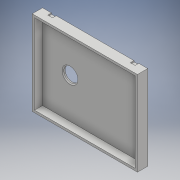
# Autodesk Inventor part: Bottom Roof
Saved by Autodesk Inventor 2017 (Build 210142000, 142)
## iProperties
Created: 2018-02-08
Part Number: Bottom Roof
Material: Generic
Document SubType Name: Modeling
Designer: Arjuna
Density: 1 g/cm^3
Appearance: Default
Author: Arjuna
## iProperties of the stored document Bottom Roof_3DPrint.ipt
Created: 2018-03-29
Part Number: Bottom Roof_3DPrint
Material: Generic
Document SubType Name: Modeling
Designer: Arjuna
Density: 1 g/cm^3
Appearance: Default
Author: Arjuna
Autodesk Inventor part; units mm, degrees
ref_plane "YZ Plane" through (0, 0, 0) normal (1, 0, 0) x (0, 1, 0)
ref_plane "XZ Plane" through (0, 0, 0) normal (0, 1, 0) x (-1, 0, 0)
ref_plane "XY Plane" through (0, 0, 0) normal (0, 0, 1) x (1, 0, 0)
sketch "Sketch1" plane through (0, 0, 0) normal (0, 1, 0) x (-1, 0, 0)
  line L0 (115, 92.5) -> (-115, 92.5)
  line L1 (-115, 92.5) -> (-115, -92.5)
  line L2 (-115, -92.5) -> (115, -92.5)
  line L3 (115, -92.5) -> (115, 92.5)
  point P0 (0, 0)
  dimension "d0" = 230
  dimension "d1" = 185
  dimension "d2" = 115
  dimension "d3" = 92.5
  constraints: 8 end point, 2 parallel, 1 horizontal, 1 perpendicular
  measures "d0" distance between parallel lines of L1 L3
  measures "d1" distance between parallel lines of L2 L0
  measures "d2" distance from line of point (0, 0) L3
  measures "d3" distance from line of point (0, 0) L2
extrude "Extrusion1" add sketch "Sketch1" along normal blind 5
sketch "Sketch2" plane through (0, 0, 0) normal (0, -1, 0) x (1, 0, 0)
  line L0 (110, 87.5) -> (-110, 87.5)
  line L1 (-110, 87.5) -> (-110, -87.5)
  line L2 (-110, -87.5) -> (110, -87.5)
  line L3 (110, -87.5) -> (110, 87.5)
  line L4 (-115, 92.5) -> (115, 92.5) projected
  line L5 (-115, -92.5) -> (-115, 92.5) projected
  line L6 (115, -92.5) -> (-115, -92.5) projected
  line L7 (115, 92.5) -> (115, -92.5) projected
  line L8 (115, 92.5) -> (-115, 92.5)
  line L9 (-115, 92.5) -> (-115, -92.5)
  line L10 (-115, -92.5) -> (115, -92.5)
  line L11 (115, -92.5) -> (115, 92.5)
  point P0 (0, 0)
  dimension "d109" = 5
  dimension "d110" = 5
  dimension "d111" = 5
  dimension "d112" = 5
  constraints: 16 end point, 4 parallel, 2 horizontal, 2 perpendicular
  measures "d109" distance between parallel lines of L2 L6
  measures "d110" distance between parallel lines of L1 L5
  measures "d111" distance between parallel lines of L4 L0
  measures "d112" distance between parallel lines of L7 L3
extrude "Extrusion2" add sketch "Sketch2" along normal blind 17.5
sketch "Sketch3" plane through (0, 5, 0) normal (0, 1, 0) x (1, 0, 0)
  circle A0 centre (-50, 0) radius 15.5
  point P0 (0, 0)
  dimension "d12" = 31
  dimension "d13" = 50
  constraints: 1 centre point
  measures "d12" diameter of A0
  measures "d13" distance of point (0, 0) A0.centre
extrude "Extrusion3" cut sketch "Sketch3" against normal through all
sketch "Sketch4" plane through (0, 5, 0) normal (0, 1, 0) x (1, 0, 0)
  circle A0 centre (-50, 0) radius 15.5 projected
  line L0 (-115, -92.5) -> (115, -92.5) projected
  line L1 (115, -92.5) -> (115, 92.5) projected
  line L2 (115, 92.5) -> (-115, 92.5) projected
  line L3 (-115, 92.5) -> (-115, -92.5) projected
  circle A1 centre (-97.5, -75) radius 7.5
  circle A2 centre (-97.5, 75) radius 7.5
  circle A3 centre (97.5, -75) radius 7.5
  circle A4 centre (97.5, 75) radius 7.5
  circle A5 centre (-97.5, -75) radius 8.5
  circle A6 centre (-97.5, 75) radius 8.5
  circle A7 centre (97.5, 75) radius 8.5
  circle A8 centre (97.5, -75) radius 8.5
  point P0 (0, 0)
  dimension "d16" = 15
  dimension "d17" = 17.5
  dimension "d18" = 17.5
  dimension "d19" = 15
  dimension "d20" = 15
  dimension "d21" = 15
  dimension "d22" = 17.5
  dimension "d23" = 17.5
  dimension "d24" = 17.5
  dimension "d25" = 17.5
  dimension "d26" = 17.5
  dimension "d27" = 17.5
  dimension "d28" = 17
  dimension "d29" = 17
  dimension "d30" = 17
  dimension "d31" = 17
  dimension "d34" = 75
  dimension "d35" = 97.5
  constraints: 8 centre point, 4 coincident
  measures "d16" diameter of A1
  measures "d17" distance from line of A1.centre L3
  measures "d18" distance from line of L0 A1.centre
  measures "d19" diameter of A2
  measures "d20" diameter of A3
  measures "d21" diameter of A4
  measures "d22" distance from line of L3 A2.centre
  measures "d23" distance from line of L2 A2.centre
  measures "d24" distance from line of L1 A4.centre
  measures "d25" distance from line of L2 A4.centre
  measures "d26" distance from line of L1 A3.centre
  measures "d27" distance from line of L0 A3.centre
  measures "d28" diameter of A5
  measures "d29" diameter of A6
  measures "d30" diameter of A7
  measures "d31" diameter of A8
  measures "d34" vertical distance of point (0, 0) A1.centre
  measures "d35" horizontal distance of point (0, 0) A1.centre
extrude "Extrusion4" [suppressed]
sketch "Sketch8" plane through (0, 5, 0) normal (0, 1, 0) x (1, 0, 0)
  circle A0 centre (-50, 0) radius 15.5 projected
  line L0 (-115, -92.5) -> (115, -92.5) projected
  line L1 (115, -92.5) -> (115, 92.5) projected
  line L2 (115, 92.5) -> (-115, 92.5) projected
  line L3 (-115, 92.5) -> (-115, -92.5) projected
  line L4 (-50, 13.5) -> (-50, -13.5)
  line L5 (-50, 13.5) -> (-115, 13.5)
  line L6 (-50, -13.5) -> (-115, -13.5)
  line L7 (-115, -13.5) -> (-115, 13.5)
  point P0 (0, 0)
  dimension "d51" = 27
  dimension "d52" = 13.5
  dimension "d62" = 31
  constraints: 8 end point, 2 perpendicular, 2 point on line, 1 collinear, 1 vertical
  measures "d51" distance of L4.start L4.end
  measures "d52" distance of A0.centre L4.start
  measures "d62" diameter of A0
extrude "Extrusion8" [suppressed]
sketch "Sketch10" plane through (-115, 5, -13.5) normal (0, 0, 1) x (1, 0, 0)
  line L0 (5, -20) -> (0, -20) projected
  line L1 (5, -5) -> (5, -20) projected
  line L2 (65, -5) -> (5, -5) projected
  line L3 (65, 0) -> (65, -5) projected
  line L4 (0, 0) -> (65, 0) projected
  line L5 (0, -20) -> (0, 0) projected
  line L6 (5, -17.5) -> (2.5, -17.5)
  line L7 (2.5, -17.5) -> (2.5, -2.5)
  line L8 (2.5, -2.5) -> (5, -2.5)
  line L9 (5, -2.5) -> (5, -17.5)
  line L10 (62.5, -5) -> (2.5, -5)
  line L11 (2.5, -5) -> (2.5, -2.5)
  line L12 (2.5, -2.5) -> (62.5, -2.5)
  line L13 (62.5, -2.5) -> (62.5, -5)
  point P0 (115, -5)
  dimension "d64" = 2.5
  dimension "d65" = 15
  dimension "d67" = 2.5
  dimension "d68" = 2.5
  dimension "d71" = 2.5
  dimension "d72" = 0
  constraints: 16 end point, 4 parallel, 2 horizontal, 2 perpendicular, 2 point on line
  measures "d64" distance of L7.end L8.end
  measures "d65" distance between parallel lines of L0 L2
  measures "d67" distance between parallel lines of L2 L12
  measures "d68" distance between parallel lines of L13 L3
  measures "d71" distance between parallel lines of L0 L6
  measures "d72" distance between parallel lines of L11 L7
extrude "Extrusion10" [suppressed]
mirror "Mirror3" [suppressed]
sketch "Sketch12" plane through (0, 5, 0) normal (0, 1, 0) x (1, 0, 0)
  line L0 (-115, 13.5) -> (-110, 13.5)
  line L1 (-110, 13.5) -> (-110, 87.5)
  line L2 (-110, 87.5) -> (110, 87.5)
  line L3 (110, 87.5) -> (110, -87.5)
  line L4 (110, -87.5) -> (-110, -87.5)
  line L5 (-110, -87.5) -> (-110, -13.5)
  line L6 (-110, -13.5) -> (-115, -13.5)
  line L7 (-115, -13.5) -> (-115, -92.5)
  line L8 (-115, -92.5) -> (115, -92.5)
  line L9 (115, -92.5) -> (115, 92.5)
  line L10 (115, 92.5) -> (-115, 92.5)
  line L11 (-115, 92.5) -> (-115, 13.5)
  line L12 (-95.5, -92.5) -> (-85, -92.5)
  line L13 (-85, -92.5) -> (-85, -90)
  line L14 (-85, -90) -> (-95.5, -90)
  line L15 (-95.5, -90) -> (-95.5, -92.5)
  line L16 (85, -92.5) -> (95.5, -92.5)
  line L17 (95.5, -92.5) -> (95.5, -90)
  line L18 (95.5, -90) -> (85, -90)
  line L19 (85, -90) -> (85, -92.5)
  line L20 (-95.5, 92.5) -> (-85, 92.5)
  line L21 (-85, 92.5) -> (-85, 90)
  line L22 (-85, 90) -> (-95.5, 90)
  line L23 (-95.5, 90) -> (-95.5, 92.5)
  line L24 (85, 92.5) -> (95.5, 92.5)
  line L25 (95.5, 92.5) -> (95.5, 90)
  line L26 (95.5, 90) -> (85, 90)
  line L27 (85, 90) -> (85, 92.5)
  point P0 (0, 0)
  point P1 (0, 0)
  dimension "d87" = 10.5
  dimension "d88" = 2.5
  dimension "d90" = 10.5
  dimension "d91" = 2.5
  dimension "d93" = 2.5
  dimension "d94" = 10.5
  dimension "d96" = 2.5
  dimension "d97" = 10.5
  dimension "d114" = 85
  dimension "d115" = 85
  dimension "d116" = 85
  dimension "d117" = 85
  dimension "d122" = 5
  dimension "d123" = 5
  dimension "d124" = 230
  dimension "d125" = 230
  dimension "d126" = 19.5
  dimension "d127" = 19.5
  dimension "d128" = 19.5
  dimension "d129" = 19.5
  dimension "d131" = 5
  constraints: 56 end point, 8 parallel, 4 horizontal, 4 perpendicular, 4 point on line
  measures "d87" distance of L14.end L13.end
  measures "d88" distance between parallel lines of L14 L12
  measures "d90" distance of L18.end L17.end
  measures "d91" distance between parallel lines of L18 L8
  measures "d93" distance between parallel lines of L20 L22
  measures "d94" distance between parallel lines of L21 L23
  measures "d96" distance between parallel lines of L10 L26
  measures "d97" distance between parallel lines of L25 L27
  measures "d114" distance from line of point (0, 0) L13
  measures "d115" distance from line of point (0, 0) L21
  measures "d116" distance from line of point (0, 0) L19
  measures "d117" distance from line of point (0, 0) L27
  measures "d122" distance between parallel lines of L1 L11
  measures "d123" distance between parallel lines of L9 L3
  measures "d124" distance of L7.end L8.end
  measures "d125" distance of L9.end L10.end
  measures "d126" distance between parallel lines of L9 L17
  measures "d127" distance between parallel lines of L9 L25
  measures "d128" distance between parallel lines of L7 L15
  measures "d129" distance between parallel lines of L11 L23
  measures "d131" distance between parallel lines of L5 L7
extrude "Extrusion12" cut sketch "Sketch12" against normal blind 8 contours L10 L21 L22 L23 | L10 L25 L26 L27 | L8 L19 L18 L17 | L15 L14 L13 L8
sketch "Sketch13" plane through (0, -17.5, 0) normal (0, -1, 0) x (1, 0, 0)
  line L0 (-110, -87.5) -> (-110, 87.5) projected
  line L1 (-110, 87.5) -> (110, 87.5) projected
  line L2 (110, 87.5) -> (110, -87.5) projected
  line L3 (110, -87.5) -> (-110, -87.5) projected
  line L4 (-115, 92.5) -> (-115, -92.5) projected
  line L5 (-115, -92.5) -> (115, -92.5) projected
  line L6 (115, -92.5) -> (115, 92.5) projected
  line L7 (115, 92.5) -> (-115, 92.5) projected
  line L8 (112.75, -90.25) -> (-112.75, -90.25)
  line L9 (-112.75, -90.25) -> (-112.75, 90.25)
  line L10 (-112.75, 90.25) -> (112.75, 90.25)
  line L11 (112.75, 90.25) -> (112.75, -90.25)
  point P0 (0, 0)
  dimension "d101" = 185
  dimension "d102" = 180.5
  dimension "d104" = 225.5
  dimension "d105" = 112.75
  dimension "d106" = 90.25
  constraints: 8 end point, 2 parallel, 1 horizontal, 1 perpendicular
  measures "d101" distance between parallel lines of L7 L5
  measures "d102" distance between parallel lines of L10 L8
  measures "d104" distance between parallel lines of L9 L11
  measures "d105" distance from line of point (0, 0) L11
  measures "d106" distance from line of point (0, 0) L8
extrude "Extrusion13" [suppressed]
fillet "Fillet1" radius 2 1 edges at (-65.5, 0, 0)
equation "\"d2\" = 0.5 * d0"
equation "\"d3\" = 0.5 * d1"
equation "\"d110\" = d109"
equation "\"d111\" = d109"
equation "\"d112\" = d109"
equation "\"d18\" = d17"
equation "\"d19\" = d16"
equation "\"d20\" = d16"
equation "\"d21\" = d16"
equation "\"d22\" = d17"
equation "\"d23\" = d22"
equation "\"d24\" = d17"
equation "\"d25\" = d24"
equation "\"d26\" = d17"
equation "\"d27\" = d26"
equation "\"d29\" = d28"
equation "\"d30\" = d28"
equation "\"d31\" = d28"
equation "\"d52\" = 0.5 * d51"
equation "\"d90\" = d87"
equation "\"d91\" = d88"
equation "\"d93\" = d88"
equation "\"d94\" = d87"
equation "\"d96\" = d88"
equation "\"d97\" = d87"
equation "\"d115\" = d114"
equation "\"d116\" = d114"
equation "\"d117\" = d114"
equation "\"d105\" = 0.5 * d104"
equation "\"d106\" = 0.5 * d102"
body "Solid1"
